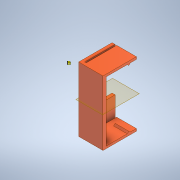
# Autodesk Inventor part: usbHubCaseTopChargingSide
Saved by Autodesk Inventor 2021.2 (Build 252289000, 289)
## iProperties
Created: 2021-02-17
Part Number: usbHubCaseTopChargingSide
Material: PC/ABS Plastic
Document SubType Name: Modeling
Designer: robst
Density: 0.357273 g/cm^3
Appearance: Smooth - Light Orange
Author: robst
Autodesk Inventor part; units mm, degrees
ref_plane "YZ Plane" through (0, 0, 0) normal (1, 0, 0) x (0, 1, 0)
ref_plane "XY Plane" through (0, 0, 0) normal (0, 0, 1) x (1, 0, 0)
sketch "Sketch1" plane through (0, 0, 0) normal (0, 0, 1) x (1, 0, 0)
  line L0 (-10.16, -26.9875) -> (10.16, -26.9875)
  line L1 (10.16, -26.9875) -> (10.16, 26.9875)
  line L2 (10.16, 26.9875) -> (-10.16, 26.9875)
  line L3 (-10.16, 26.9875) -> (-10.16, -26.9875)
  line L4 (-10.16, -26.9875) -> (10.16, 26.9875) construction
  line L5 (10.16, -26.9875) -> (-10.16, 26.9875) construction
  point P0 (0, 0)
  dimension "d0" = 53.975
  dimension "d1" = 20.32
  constraints: 12 end point, 2 midpoint, 2 parallel, 1 horizontal, 1 perpendicular
  measures "d0" distance of L2.end L0.start
  measures "d1" distance of L1.end L2.end
extrude "Extrusion1" add sketch "Sketch1" against normal blind 2.54
sketch "Sketch8" plane through (0, 0, -2.54) normal (0, 0, -1) x (-1, 0, 0)
  line L0 (-10.16, 26.9875) -> (-10.16, -26.9875) projected
  line L1 (10.16, -26.9875) -> (10.16, 26.9875) projected
  line L2 (-10.16, 26.9875) -> (10.16, 26.9875)
  line L3 (10.16, 26.9875) -> (10.16, 25.0825)
  line L4 (10.16, 25.0825) -> (-10.16, 25.0825)
  line L5 (-10.16, 25.0825) -> (-10.16, 26.9875)
  line L6 (-10.16, -26.9875) -> (10.16, -26.9875)
  line L7 (10.16, -26.9875) -> (10.16, -25.0825)
  line L8 (10.16, -25.0825) -> (-10.16, -25.0825)
  line L9 (-10.16, -25.0825) -> (-10.16, -26.9875)
  line L10 (10.16, 25.0825) -> (7.62, 25.0825)
  line L11 (7.62, 25.0825) -> (7.62, 9.525)
  line L12 (7.62, 9.525) -> (10.16, 9.525)
  line L13 (10.16, 9.525) -> (10.16, 25.0825)
  line L14 (10.16, -25.0825) -> (7.62, -25.0825)
  line L15 (7.62, -25.0825) -> (7.62, -9.525)
  line L16 (7.62, -9.525) -> (10.16, -9.525)
  line L17 (10.16, -9.525) -> (10.16, -25.0825)
  point P0 (0, 0)
  point P1 (10.16, -9.525)
  point P2 (10.16, 9.525)
  dimension "d32" = 1.905
  dimension "d33" = 1.905
  dimension "d34" = 2.54
  dimension "d35" = 15.5575
  dimension "d36" = 15.5575
  dimension "d37" = 2.54
  dimension "d54" = 19.05
  constraints: 32 end point, 8 parallel, 4 horizontal, 4 perpendicular, 2 point on line
  measures "d32" distance between parallel lines of L4 L2
  measures "d33" distance between parallel lines of L8 L6
  measures "d34" distance between parallel lines of L11 L1
  measures "d35" distance between parallel lines of L12 L4
  measures "d36" distance between parallel lines of L16 L8
  measures "d37" distance between parallel lines of L1 L15
  measures "d54" distance between parallel lines of L16 L12
extrude "Extrusion7" add sketch "Sketch8" along normal blind 25.4 contours L2 L1 L4 L0 | L8 L1 L6 L0 | L4 L1 L12 L11 | L15 L16 L1 L8
sketch "Sketch10" plane through (0, 0, -2.54) normal (0, 0, -1) x (-1, 0, 0)
  line L0 (7.62, 25.0825) -> (7.62, 9.525) projected
  line L1 (7.62, 9.525) -> (10.16, 9.525)
  line L2 (10.16, 9.525) -> (10.16, -9.525)
  line L3 (10.16, -9.525) -> (7.62, -9.525)
  line L4 (7.62, -9.525) -> (7.62, 9.525)
  point P0 (0, 0)
  constraints: 8 end point, 2 parallel, 1 horizontal, 1 perpendicular
extrude "Extrusion8" add sketch "Sketch10" along normal blind 6.096
sketch "Sketch11" plane through (10.16, -26.9875, 0) normal (1, 0, 0) x (0, 0, -1)
  line L0 (2.54, 1.905) -> (27.94, 1.905) projected
  line L1 (2.54, 52.07) -> (27.94, 52.07) projected
  line L2 (20.32, 1.905) -> (21.59, 3.175)
  line L3 (21.59, 3.175) -> (22.86, 1.905)
  line L4 (2.54, 1.905) -> (27.94, 1.905) projected
  line L5 (27.94, 17.4625) -> (27.94, 1.905) projected
  line L6 (20.32, 1.905) -> (22.86, 1.905)
  line L7 (0, 26.9875) -> (27.94, 26.9875) construction
  line L8 (2.54, 52.07) -> (27.94, 52.07)
  line L9 (20.32, 52.07) -> (21.59, 50.8)
  line L10 (21.59, 50.8) -> (22.86, 52.07)
  point P0 (22.86, 52.07)
  point P1 (20.32, 52.07)
  dimension "d42" = 90
  dimension "d43" = 135
  dimension "d44" = 1.27
  dimension "d45" = 6.35
  constraints: 14 end point, 3 point on line, 3 symmetric about line, 1 collinear, 1 horizontal
  measures "d42" angle of L3 L2
  measures "d43" angle of L3 L0
  measures "d44" distance from line of L2.end L0
  measures "d45" distance from line of L2.end L5
extrude "Extrusion9" add sketch "Sketch11" against normal up to surface (17.78 mm away)
sketch "Sketch12" plane through (-10.16, 26.9875, 0) normal (0, 1, 0) x (1, 0, 0)
  line L0 (2.54, 2.54) -> (2.54, 20.32) projected
  line L1 (2.54, 22.86) -> (2.54, 27.94) projected
  line L2 (2.54, 2.54) -> (20.32, 2.54) projected
  line L3 (2.54, 2.54) -> (3.81, 2.54)
  line L4 (3.81, 2.54) -> (3.81, 27.94)
  line L5 (3.81, 27.94) -> (2.54, 27.94)
  line L6 (2.54, 27.94) -> (2.54, 2.54)
  point P0 (10.16, 0)
  point P1 (2.54, 22.86)
  point P2 (2.54, 20.32)
  point P3 (3.81, 2.54)
  dimension "d48" = 1.27
  constraints: 8 end point, 2 parallel, 1 horizontal, 1 perpendicular
  measures "d48" distance between parallel lines of L1 L4
extrude "Extrusion10" cut sketch "Sketch12" against normal through all
sketch "Sketch16" plane through (0, 0, -2.54) normal (0, 0, -1) x (-1, 0, 0)
  line L0 (7.62, -9.525) -> (7.62, -26.9875) projected
  line L1 (-10.16, 25.0825) -> (-10.16, -25.0825) projected
  line L2 (-10.16, -26.9875) -> (6.35, -26.9875) projected
  line L3 (6.35, 26.9875) -> (-10.16, 26.9875) projected
  line L4 (-10.16, 26.9875) -> (10.16, 26.9875) construction
  line L5 (-0.762, 26.9875) -> (-0.762, -26.9875) construction
  line L6 (10.16, -26.9875) -> (-10.16, -26.9875) construction
  spline S0 degree 2 poles (-4.6934, -4.0246) (-4.4464, -4.0246) (-4.0018, -4.2006) (-3.8475, -4.358) knots 0 0 0 1 2 2 2
  spline S1 degree 2 poles (-3.8475, -4.358) (-3.6529, -4.5556) (-3.4523, -5.0898) (-3.4523, -5.4973) knots 0 0 0 1 2 2 2
  line L7 (-3.4523, -5.4973) -> (-3.4523, -5.9265)
  line L8 (-3.4523, -5.9265) -> (-2.032, -5.9265)
  line L9 (-2.032, -5.9265) -> (-2.032, -6.4328)
  line L10 (-2.032, -6.4328) -> (-5.842, -6.4328)
  line L11 (-5.842, -6.4328) -> (-5.842, -5.4757)
  spline S2 degree 2 poles (-5.842, -5.4757) (-5.842, -5.1361) (-5.7308, -4.6606) (-5.6043, -4.4784) knots 0 0 0 1 2 2 2
  spline S3 degree 2 poles (-5.6043, -4.4784) (-5.4591, -4.2654) (-5.0115, -4.0246) (-4.6934, -4.0246) knots 0 0 0 1 2 2 2
  spline S4 degree 2 poles (-4.678, -4.5525) (-4.8756, -4.5525) (-5.1658, -4.6884) (-5.2585, -4.8273) knots 0 0 0 1 2 2 2
  spline S5 degree 2 poles (-5.2585, -4.8273) (-5.3387, -4.9478) (-5.4036, -5.2689) (-5.4036, -5.5066) knots 0 0 0 1 2 2 2
  line L12 (-5.4036, -5.5066) -> (-5.4036, -5.9265)
  line L13 (-5.4036, -5.9265) -> (-3.8845, -5.9265)
  line L14 (-3.8845, -5.9265) -> (-3.8845, -5.5807)
  spline S6 degree 2 poles (-3.8845, -5.5807) (-3.8845, -5.2719) (-3.9833, -4.8922) (-4.113, -4.7687) knots 0 0 0 1 2 2 2
  spline S7 degree 2 poles (-4.113, -4.7687) (-4.2272, -4.6544) (-4.4958, -4.5525) (-4.678, -4.5525) knots 0 0 0 1 2 2 2
  line L15 (-5.842, -0.7796) -> (-2.032, -2.0918)
  line L16 (-2.032, -2.0918) -> (-2.032, -2.6383)
  line L17 (-2.032, -2.6383) -> (-5.842, -3.9505)
  line L18 (-5.842, -3.9505) -> (-5.842, -3.4071)
  line L19 (-5.842, -3.4071) -> (-2.6773, -2.3511)
  line L20 (-2.6773, -2.3511) -> (-5.842, -1.2952)
  line L21 (-5.842, -1.2952) -> (-5.842, -0.7796)
  line L22 (-3.4677, 0.9154) -> (-3.4677, -0.5264)
  line L23 (-3.4677, -0.5264) -> (-3.9308, -0.5264)
  line L24 (-3.9308, -0.5264) -> (-3.9308, 0.9154)
  line L25 (-3.9308, 0.9154) -> (-3.4677, 0.9154)
  spline S8 degree 2 poles (-3.937, 3.793) (-2.9119, 3.793) (-1.9517, 3.1971) (-1.9517, 2.5765) knots 0 0 0 1 2 2 2
  spline S9 degree 2 poles (-1.9517, 2.5765) (-1.9517, 1.9467) (-2.9305, 1.357) (-3.9339, 1.357) knots 0 0 0 1 2 2 2
  spline S10 degree 2 poles (-3.9339, 1.357) (-4.9651, 1.357) (-5.9192, 1.9529) (-5.9192, 2.5765) knots 0 0 0 1 2 2 2
  spline S11 degree 2 poles (-5.9192, 2.5765) (-5.9192, 3.2033) (-4.9312, 3.793) (-3.937, 3.793) knots 0 0 0 1 2 2 2
  spline S12 degree 2 poles (-2.7761, 3.1385) (-2.9644, 3.2126) (-3.5449, 3.2743) (-3.937, 3.2743) knots 0 0 0 1 2 2 2
  spline S13 degree 2 poles (-3.937, 3.2743) (-4.3291, 3.2743) (-4.9065, 3.2126) (-5.101, 3.1354) knots 0 0 0 1 2 2 2
  spline S14 degree 2 poles (-5.101, 3.1354) (-5.2955, 3.0582) (-5.4962, 2.7896) (-5.4962, 2.5765) knots 0 0 0 1 2 2 2
  spline S15 degree 2 poles (-5.4962, 2.5765) (-5.4962, 2.3635) (-5.2955, 2.0887) (-5.0948, 2.0084) knots 0 0 0 1 2 2 2
  spline S16 degree 2 poles (-5.0948, 2.0084) (-4.9003, 1.9312) (-4.3075, 1.8757) (-3.9339, 1.8757) knots 0 0 0 1 2 2 2
  spline S17 degree 2 poles (-3.9339, 1.8757) (-3.5325, 1.8757) (-2.9953, 1.9251) (-2.7854, 2.0053) knots 0 0 0 1 2 2 2
  spline S18 degree 2 poles (-2.7854, 2.0053) (-2.5878, 2.0794) (-2.3747, 2.3542) (-2.3747, 2.5765) knots 0 0 0 1 2 2 2
  spline S19 degree 2 poles (-2.3747, 2.5765) (-2.3747, 2.7865) (-2.5754, 3.0613) (-2.7761, 3.1385) knots 0 0 0 1 2 2 2
  line L26 (-3.3411, 6.7323) -> (-3.3411, 6.2785)
  line L27 (-3.3411, 6.2785) -> (-2.032, 6.2785)
  line L28 (-2.032, 6.2785) -> (-2.032, 5.7876)
  line L29 (-2.032, 5.7876) -> (-3.3411, 5.7876)
  line L30 (-3.3411, 5.7876) -> (-3.3411, 4.1049)
  line L31 (-3.3411, 4.1049) -> (-3.8783, 4.1049)
  line L32 (-3.8783, 4.1049) -> (-5.842, 5.8092)
  line L33 (-5.842, 5.8092) -> (-5.842, 6.2785)
  line L34 (-5.842, 6.2785) -> (-3.7517, 6.2785)
  line L35 (-3.7517, 6.2785) -> (-3.7517, 6.7323)
  line L36 (-3.7517, 6.7323) -> (-3.3411, 6.7323)
  line L37 (-3.7517, 5.7876) -> (-5.2399, 5.7876)
  line L38 (-5.2399, 5.7876) -> (-3.7517, 4.5062)
  line L39 (-3.7517, 4.5062) -> (-3.7517, 5.7876)
  spline S20 degree 2 poles (4.4171, -14.1378) (4.4171, -14.5083) (4.1671, -15.135) (3.917, -15.3635) knots 0 0 0 1 2 2 2
  spline S21 degree 2 poles (3.917, -15.3635) (3.67, -15.592) (2.929, -15.8421) (2.4473, -15.8421) knots 0 0 0 1 2 2 2
  spline S22 degree 2 poles (2.4473, -15.8421) (1.9687, -15.8421) (1.2586, -15.5982) (0.9962, -15.3666) knots 0 0 0 1 2 2 2
  spline S23 degree 2 poles (0.9962, -15.3666) (0.7399, -15.1381) (0.4713, -14.5144) (0.4713, -14.1285) knots 0 0 0 1 2 2 2
  spline S24 degree 2 poles (0.4713, -14.1285) (0.4713, -13.9371) (0.5269, -13.6005) (0.5701, -13.4585) knots 0 0 0 1 2 2 2
  spline S25 degree 2 poles (0.5701, -13.4585) (0.6102, -13.335) (0.7245, -13.0787) (0.7924, -12.9521) knots 0 0 0 1 2 2 2
  line L40 (0.7924, -12.9521) -> (1.4037, -12.9521)
  line L41 (1.4037, -12.9521) -> (1.4037, -12.9923)
  spline S26 degree 2 poles (1.4037, -12.9923) (1.342, -13.0602) (1.1691, -13.2702) (1.0857, -13.4215) knots 0 0 0 1 2 2 2
  spline S27 degree 2 poles (1.0857, -13.4215) (1.0054, -13.5666) (0.9035, -13.9093) (0.9035, -14.1316) knots 0 0 0 1 2 2 2
  spline S28 degree 2 poles (0.9035, -14.1316) (0.9035, -14.3755) (1.1042, -14.8108) (1.2957, -14.9745) knots 0 0 0 1 2 2 2
  spline S29 degree 2 poles (1.2957, -14.9745) (1.4902, -15.135) (2.0799, -15.3141) (2.4473, -15.3141) knots 0 0 0 1 2 2 2
  spline S30 degree 2 poles (2.4473, -15.3141) (2.8394, -15.3141) (3.4044, -15.1258) (3.5989, -14.9621) knots 0 0 0 1 2 2 2
  spline S31 degree 2 poles (3.5989, -14.9621) (3.7873, -14.8016) (3.9787, -14.3724) (3.9787, -14.1316) knots 0 0 0 1 2 2 2
  spline S32 degree 2 poles (3.9787, -14.1316) (3.9787, -13.9124) (3.8707, -13.5388) (3.7904, -13.3937) knots 0 0 0 1 2 2 2
  spline S33 degree 2 poles (3.7904, -13.3937) (3.7101, -13.2547) (3.5434, -13.0479) (3.4847, -12.9892) knots 0 0 0 1 2 2 2
  line L42 (3.4847, -12.9892) -> (3.4847, -12.9521)
  line L43 (3.4847, -12.9521) -> (4.0899, -12.9521)
  spline S34 degree 2 poles (4.0899, -12.9521) (4.1485, -13.0787) (4.2566, -13.301) (4.306, -13.4585) knots 0 0 0 1 2 2 2
  spline S35 degree 2 poles (4.306, -13.4585) (4.3616, -13.6252) (4.4171, -13.9093) (4.4171, -14.1378) knots 0 0 0 1 2 2 2
  line L44 (4.3492, -10.2722) -> (4.3492, -10.7538)
  line L45 (4.3492, -10.7538) -> (2.719, -10.7538)
  spline S36 degree 2 poles (2.719, -10.7538) (2.5214, -10.7538) (2.1818, -10.7909) (2.0799, -10.8465) knots 0 0 0 1 2 2 2
  spline S37 degree 2 poles (2.0799, -10.8465) (1.9718, -10.9051) (1.8669, -11.1151) (1.8669, -11.2941) knots 0 0 0 1 2 2 2
  spline S38 degree 2 poles (1.8669, -11.2941) (1.8669, -11.4732) (2.0583, -11.853) (2.2127, -12.0352) knots 0 0 0 1 2 2 2
  line L46 (2.2127, -12.0352) -> (4.3492, -12.0352)
  line L47 (4.3492, -12.0352) -> (4.3492, -12.5168)
  line L48 (4.3492, -12.5168) -> (0.3694, -12.5168)
  line L49 (0.3694, -12.5168) -> (0.3694, -12.0352)
  line L50 (0.3694, -12.0352) -> (1.8082, -12.0352)
  spline S39 degree 2 poles (1.8082, -12.0352) (1.6137, -11.819) (1.4099, -11.4022) (1.4099, -11.1676) knots 0 0 0 1 2 2 2
  spline S40 degree 2 poles (1.4099, -11.1676) (1.4099, -10.7477) (1.9657, -10.2722) (2.4936, -10.2722) knots 0 0 0 1 2 2 2
  line L51 (2.4936, -10.2722) -> (4.3492, -10.2722)
  spline S41 degree 2 poles (4.0466, -8.0029) (4.0899, -8.0615) (4.2442, -8.2591) (4.2906, -8.3517) knots 0 0 0 1 2 2 2
  spline S42 degree 2 poles (4.2906, -8.3517) (4.3585, -8.4783) (4.4295, -8.7161) (4.4295, -8.9322) knots 0 0 0 1 2 2 2
  spline S43 degree 2 poles (4.4295, -8.9322) (4.4295, -9.1082) (4.2967, -9.4262) (4.1763, -9.5466) knots 0 0 0 1 2 2 2
  spline S44 degree 2 poles (4.1763, -9.5466) (4.059, -9.6609) (3.7132, -9.7998) (3.5218, -9.7998) knots 0 0 0 1 2 2 2
  spline S45 degree 2 poles (3.5218, -9.7998) (3.2254, -9.7998) (2.8055, -9.5497) (2.685, -9.278) knots 0 0 0 1 2 2 2
  spline S46 degree 2 poles (2.685, -9.278) (2.5739, -9.0372) (2.4905, -8.3826) (2.4689, -8.0029) knots 0 0 0 1 2 2 2
  line L52 (2.4689, -8.0029) -> (2.3763, -8.0029)
  spline S47 degree 2 poles (2.3763, -8.0029) (2.2096, -8.0029) (2.0027, -8.1047) (1.944, -8.1974) knots 0 0 0 1 2 2 2
  spline S48 degree 2 poles (1.944, -8.1974) (1.8854, -8.29) (1.8483, -8.5555) (1.8483, -8.6975) knots 0 0 0 1 2 2 2
  spline S49 degree 2 poles (1.8483, -8.6975) (1.8483, -8.8643) (1.9471, -9.315) (2.0428, -9.5404) knots 0 0 0 1 2 2 2
  line L53 (2.0428, -9.5404) -> (2.0428, -9.5682)
  line L54 (2.0428, -9.5682) -> (1.5519, -9.5682)
  spline S50 degree 2 poles (1.5519, -9.5682) (1.5149, -9.4355) (1.4222, -8.9384) (1.4222, -8.6945) knots 0 0 0 1 2 2 2
  spline S51 degree 2 poles (1.4222, -8.6945) (1.4222, -8.3981) (1.5149, -7.9936) (1.6353, -7.833) knots 0 0 0 1 2 2 2
  spline S52 degree 2 poles (1.6353, -7.833) (1.7526, -7.6756) (2.1262, -7.5212) (2.3948, -7.5212) knots 0 0 0 1 2 2 2
  line L55 (2.3948, -7.5212) -> (4.3492, -7.5212)
  line L56 (4.3492, -7.5212) -> (4.3492, -8.0029)
  line L57 (4.3492, -8.0029) -> (4.0466, -8.0029)
  line L58 (3.6453, -8.0029) -> (2.8518, -8.0029)
  spline S53 degree 2 poles (2.8518, -8.0029) (2.8672, -8.1758) (2.9197, -8.6975) (2.9691, -8.8612) knots 0 0 0 1 2 2 2
  spline S54 degree 2 poles (2.9691, -8.8612) (3.0278, -9.0526) (3.2717, -9.3027) (3.4878, -9.3027) knots 0 0 0 1 2 2 2
  spline S55 degree 2 poles (3.4878, -9.3027) (3.7348, -9.3027) (3.9849, -9.0248) (3.9849, -8.7593) knots 0 0 0 1 2 2 2
  spline S56 degree 2 poles (3.9849, -8.7593) (3.9849, -8.5339) (3.7904, -8.1634) (3.6453, -8.0029) knots 0 0 0 1 2 2 2
  line L59 (2.0058, -5.3291) -> (2.0058, -5.3538)
  spline S57 degree 2 poles (2.0058, -5.3538) (1.9904, -5.4093) (1.9842, -5.5297) (1.9842, -5.6131) knots 0 0 0 1 2 2 2
  spline S58 degree 2 poles (1.9842, -5.6131) (1.9842, -5.8076) (2.154, -6.1905) (2.3207, -6.3634) knots 0 0 0 1 2 2 2
  line L60 (2.3207, -6.3634) -> (4.3492, -6.3634)
  line L61 (4.3492, -6.3634) -> (4.3492, -6.845)
  line L62 (4.3492, -6.845) -> (1.4902, -6.845)
  line L63 (1.4902, -6.845) -> (1.4902, -6.3634)
  line L64 (1.4902, -6.3634) -> (1.9163, -6.3634)
  spline S59 degree 2 poles (1.9163, -6.3634) (1.6816, -6.1009) (1.4902, -5.7088) (1.4902, -5.5236) knots 0 0 0 1 2 2 2
  spline S60 degree 2 poles (1.4902, -5.5236) (1.4902, -5.4495) (1.4963, -5.3754) (1.5056, -5.3291) knots 0 0 0 1 2 2 2
  line L65 (1.5056, -5.3291) -> (2.0058, -5.3291)
  spline S61 degree 2 poles (4.8062, -4.8536) (4.8278, -4.8042) (4.8957, -4.6158) (4.9235, -4.4954) knots 0 0 0 1 2 2 2
  spline S62 degree 2 poles (4.9235, -4.4954) (4.9575, -4.3627) (4.9976, -4.1373) (4.9976, -4.0045) knots 0 0 0 1 2 2 2
  spline S63 degree 2 poles (4.9976, -4.0045) (4.9976, -3.7822) (4.8803, -3.4735) (4.7753, -3.387) knots 0 0 0 1 2 2 2
  spline S64 degree 2 poles (4.7753, -3.387) (4.6703, -3.3036) (4.3955, -3.2388) (4.2195, -3.2388) knots 0 0 0 1 2 2 2
  line L66 (4.2195, -3.2388) -> (3.9695, -3.2388)
  spline S65 degree 2 poles (3.9695, -3.2388) (4.1393, -3.4333) (4.2998, -3.8069) (4.2998, -4.0879) knots 0 0 0 1 2 2 2
  spline S66 degree 2 poles (4.2998, -4.0879) (4.2998, -4.5757) (3.5742, -5.1531) (2.8919, -5.1531) knots 0 0 0 1 2 2 2
  spline S67 degree 2 poles (2.8919, -5.1531) (2.5368, -5.1531) (1.9873, -4.9524) (1.7928, -4.7857) knots 0 0 0 1 2 2 2
  spline S68 degree 2 poles (1.7928, -4.7857) (1.6106, -4.6251) (1.4099, -4.1836) (1.4099, -3.9489) knots 0 0 0 1 2 2 2
  spline S69 degree 2 poles (1.4099, -3.9489) (1.4099, -3.7266) (1.5149, -3.4024) (1.6106, -3.2388) knots 0 0 0 1 2 2 2
  line L67 (1.6106, -3.2388) -> (1.4902, -3.211)
  line L68 (1.4902, -3.211) -> (1.4902, -2.7572)
  line L69 (1.4902, -2.7572) -> (4.0219, -2.7572)
  spline S70 degree 2 poles (4.0219, -2.7572) (4.7506, -2.7572) (5.4298, -3.3901) (5.4298, -4.0416) knots 0 0 0 1 2 2 2
  spline S71 degree 2 poles (5.4298, -4.0416) (5.4298, -4.2515) (5.3619, -4.6899) (5.3063, -4.8783) knots 0 0 0 1 2 2 2
  line L70 (5.3063, -4.8783) -> (4.8062, -4.8783)
  line L71 (4.8062, -4.8783) -> (4.8062, -4.8536)
  line L72 (3.5742, -3.2388) -> (2.0027, -3.2388)
  spline S72 degree 2 poles (2.0027, -3.2388) (1.9163, -3.4179) (1.8422, -3.7205) (1.8422, -3.8718) knots 0 0 0 1 2 2 2
  spline S73 degree 2 poles (1.8422, -3.8718) (1.8422, -4.2361) (2.3794, -4.656) (2.8826, -4.656) knots 0 0 0 1 2 2 2
  spline S74 degree 2 poles (2.8826, -4.656) (3.3581, -4.656) (3.8552, -4.338) (3.8552, -3.9798) knots 0 0 0 1 2 2 2
  spline S75 degree 2 poles (3.8552, -3.9798) (3.8552, -3.7915) (3.707, -3.3963) (3.5742, -3.2388) knots 0 0 0 1 2 2 2
  line L73 (4.3492, -1.5685) -> (4.3492, -2.0501)
  line L74 (4.3492, -2.0501) -> (1.4902, -2.0501)
  line L75 (1.4902, -2.0501) -> (1.4902, -1.5685)
  line L76 (1.4902, -1.5685) -> (4.3492, -1.5685)
  line L77 (1.0147, -1.5345) -> (1.0147, -2.081)
  line L78 (1.0147, -2.081) -> (0.5145, -2.081)
  line L79 (0.5145, -2.081) -> (0.5145, -1.5345)
  line L80 (0.5145, -1.5345) -> (1.0147, -1.5345)
  line L81 (4.3492, 1.3832) -> (4.3492, 0.9016)
  line L82 (4.3492, 0.9016) -> (2.719, 0.9016)
  spline S76 degree 2 poles (2.719, 0.9016) (2.5214, 0.9016) (2.1818, 0.8645) (2.0799, 0.8089) knots 0 0 0 1 2 2 2
  spline S77 degree 2 poles (2.0799, 0.8089) (1.9718, 0.7503) (1.8669, 0.5403) (1.8669, 0.3612) knots 0 0 0 1 2 2 2
  spline S78 degree 2 poles (1.8669, 0.3612) (1.8669, 0.1822) (2.0583, -0.1976) (2.2127, -0.3798) knots 0 0 0 1 2 2 2
  line L83 (2.2127, -0.3798) -> (4.3492, -0.3798)
  line L84 (4.3492, -0.3798) -> (4.3492, -0.8614)
  line L85 (4.3492, -0.8614) -> (1.4902, -0.8614)
  line L86 (1.4902, -0.8614) -> (1.4902, -0.3798)
  line L87 (1.4902, -0.3798) -> (1.8082, -0.3798)
  spline S79 degree 2 poles (1.8082, -0.3798) (1.6137, -0.1636) (1.4099, 0.2532) (1.4099, 0.4878) knots 0 0 0 1 2 2 2
  spline S80 degree 2 poles (1.4099, 0.4878) (1.4099, 0.9077) (1.9657, 1.3832) (2.4936, 1.3832) knots 0 0 0 1 2 2 2
  line L88 (2.4936, 1.3832) -> (4.3492, 1.3832)
  spline S81 degree 2 poles (4.8062, 2.1613) (4.8278, 2.2107) (4.8957, 2.399) (4.9235, 2.5194) knots 0 0 0 1 2 2 2
  spline S82 degree 2 poles (4.9235, 2.5194) (4.9575, 2.6522) (4.9976, 2.8776) (4.9976, 3.0103) knots 0 0 0 1 2 2 2
  spline S83 degree 2 poles (4.9976, 3.0103) (4.9976, 3.2326) (4.8803, 3.5414) (4.7753, 3.6278) knots 0 0 0 1 2 2 2
  spline S84 degree 2 poles (4.7753, 3.6278) (4.6703, 3.7112) (4.3955, 3.776) (4.2195, 3.776) knots 0 0 0 1 2 2 2
  line L89 (4.2195, 3.776) -> (3.9695, 3.776)
  spline S85 degree 2 poles (3.9695, 3.776) (4.1393, 3.5815) (4.2998, 3.2079) (4.2998, 2.927) knots 0 0 0 1 2 2 2
  spline S86 degree 2 poles (4.2998, 2.927) (4.2998, 2.4391) (3.5742, 1.8618) (2.8919, 1.8618) knots 0 0 0 1 2 2 2
  spline S87 degree 2 poles (2.8919, 1.8618) (2.5368, 1.8618) (1.9873, 2.0625) (1.7928, 2.2292) knots 0 0 0 1 2 2 2
  spline S88 degree 2 poles (1.7928, 2.2292) (1.6106, 2.3897) (1.4099, 2.8313) (1.4099, 3.0659) knots 0 0 0 1 2 2 2
  spline S89 degree 2 poles (1.4099, 3.0659) (1.4099, 3.2882) (1.5149, 3.6124) (1.6106, 3.776) knots 0 0 0 1 2 2 2
  line L90 (1.6106, 3.776) -> (1.4902, 3.8038)
  line L91 (1.4902, 3.8038) -> (1.4902, 4.2577)
  line L92 (1.4902, 4.2577) -> (4.0219, 4.2577)
  spline S90 degree 2 poles (4.0219, 4.2577) (4.7506, 4.2577) (5.4298, 3.6247) (5.4298, 2.9733) knots 0 0 0 1 2 2 2
  spline S91 degree 2 poles (5.4298, 2.9733) (5.4298, 2.7633) (5.3619, 2.3249) (5.3063, 2.1366) knots 0 0 0 1 2 2 2
  line L93 (5.3063, 2.1366) -> (4.8062, 2.1366)
  line L94 (4.8062, 2.1366) -> (4.8062, 2.1613)
  line L95 (3.5742, 3.776) -> (2.0027, 3.776)
  spline S92 degree 2 poles (2.0027, 3.776) (1.9163, 3.597) (1.8422, 3.2944) (1.8422, 3.1431) knots 0 0 0 1 2 2 2
  spline S93 degree 2 poles (1.8422, 3.1431) (1.8422, 2.7788) (2.3794, 2.3589) (2.8826, 2.3589) knots 0 0 0 1 2 2 2
  spline S94 degree 2 poles (2.8826, 2.3589) (3.3581, 2.3589) (3.8552, 2.6769) (3.8552, 3.035) knots 0 0 0 1 2 2 2
  spline S95 degree 2 poles (3.8552, 3.035) (3.8552, 3.2234) (3.707, 3.6186) (3.5742, 3.776) knots 0 0 0 1 2 2 2
  spline S96 degree 2 poles (4.4171, 7.691) (4.4171, 7.2773) (4.2442, 6.6968) (4.1207, 6.4406) knots 0 0 0 1 2 2 2
  line L96 (4.1207, 6.4406) -> (3.4847, 6.4406)
  line L97 (3.4847, 6.4406) -> (3.4847, 6.4776)
  spline S97 degree 2 poles (3.4847, 6.4776) (3.7194, 6.7277) (3.9787, 7.3606) (3.9787, 7.654) knots 0 0 0 1 2 2 2
  spline S98 degree 2 poles (3.9787, 7.654) (3.9787, 8.0739) (3.6298, 8.503) (3.3427, 8.503) knots 0 0 0 1 2 2 2
  spline S99 degree 2 poles (3.3427, 8.503) (3.1142, 8.503) (2.8302, 8.2776) (2.7591, 8.0337) knots 0 0 0 1 2 2 2
  spline S100 degree 2 poles (2.7591, 8.0337) (2.7097, 7.8577) (2.6418, 7.5644) (2.5862, 7.3452) knots 0 0 0 1 2 2 2
  spline S101 degree 2 poles (2.5862, 7.3452) (2.5338, 7.1476) (2.3763, 6.8358) (2.2497, 6.7154) knots 0 0 0 1 2 2 2
  spline S102 degree 2 poles (2.2497, 6.7154) (2.1231, 6.598) (1.7835, 6.4684) (1.5612, 6.4684) knots 0 0 0 1 2 2 2
  spline S103 degree 2 poles (1.5612, 6.4684) (1.0981, 6.4684) (0.4713, 7.1908) (0.4713, 7.7497) knots 0 0 0 1 2 2 2
  spline S104 degree 2 poles (0.4713, 7.7497) (0.4713, 8.0708) (0.5979, 8.6389) (0.7183, 8.8828) knots 0 0 0 1 2 2 2
  line L98 (0.7183, 8.8828) -> (1.3234, 8.8828)
  line L99 (1.3234, 8.8828) -> (1.3234, 8.8457)
  spline S105 degree 2 poles (1.3234, 8.8457) (1.1567, 8.6636) (0.9097, 8.0955) (0.9097, 7.7836) knots 0 0 0 1 2 2 2
  spline S106 degree 2 poles (0.9097, 7.7836) (0.9097, 7.4317) (1.2401, 6.9963) (1.5087, 6.9963) knots 0 0 0 1 2 2 2
  spline S107 degree 2 poles (1.5087, 6.9963) (1.7495, 6.9963) (2.0367, 7.2526) (2.1015, 7.4934) knots 0 0 0 1 2 2 2
  spline S108 degree 2 poles (2.1015, 7.4934) (2.1447, 7.654) (2.2559, 8.1202) (2.3022, 8.2746) knots 0 0 0 1 2 2 2
  spline S109 degree 2 poles (2.3022, 8.2746) (2.4226, 8.6667) (2.9073, 9.031) (3.2624, 9.031) knots 0 0 0 1 2 2 2
  spline S110 degree 2 poles (3.2624, 9.031) (3.4878, 9.031) (3.9201, 8.8488) (4.0713, 8.6852) knots 0 0 0 1 2 2 2
  spline S111 degree 2 poles (4.0713, 8.6852) (4.2381, 8.503) (4.4171, 8.0399) (4.4171, 7.691) knots 0 0 0 1 2 2 2
  line L100 (4.3492, 10.0005) -> (4.3492, 9.5188)
  line L101 (4.3492, 9.5188) -> (1.4902, 9.5188)
  line L102 (1.4902, 9.5188) -> (1.4902, 10.0005)
  line L103 (1.4902, 10.0005) -> (4.3492, 10.0005)
  line L104 (1.0147, 10.0344) -> (1.0147, 9.4879)
  line L105 (1.0147, 9.4879) -> (0.5145, 9.4879)
  line L106 (0.5145, 9.4879) -> (0.5145, 10.0344)
  line L107 (0.5145, 10.0344) -> (1.0147, 10.0344)
  line L108 (4.3492, 12.9058) -> (4.3492, 12.4242)
  line L109 (4.3492, 12.4242) -> (4.059, 12.4242)
  spline S112 degree 2 poles (4.059, 12.4242) (4.1516, 12.313) (4.2751, 12.1494) (4.3276, 12.0382) knots 0 0 0 1 2 2 2
  spline S113 degree 2 poles (4.3276, 12.0382) (4.377, 11.9364) (4.4295, 11.7171) (4.4295, 11.572) knots 0 0 0 1 2 2 2
  spline S114 degree 2 poles (4.4295, 11.572) (4.4295, 11.3374) (4.235, 10.9422) (4.0466, 10.8032) knots 0 0 0 1 2 2 2
  spline S115 degree 2 poles (4.0466, 10.8032) (3.8583, 10.6643) (3.3025, 10.5099) (2.9413, 10.5099) knots 0 0 0 1 2 2 2
  spline S116 degree 2 poles (2.9413, 10.5099) (2.5646, 10.5099) (2.0151, 10.7044) (1.8082, 10.8742) knots 0 0 0 1 2 2 2
  spline S117 degree 2 poles (1.8082, 10.8742) (1.6229, 11.0317) (1.4099, 11.4732) (1.4099, 11.7171) knots 0 0 0 1 2 2 2
  spline S118 degree 2 poles (1.4099, 11.7171) (1.4099, 11.9302) (1.5056, 12.2482) (1.6044, 12.4242) knots 0 0 0 1 2 2 2
  line L110 (1.6044, 12.4242) -> (0.3694, 12.4242)
  line L111 (0.3694, 12.4242) -> (0.3694, 12.9058)
  line L112 (0.3694, 12.9058) -> (4.3492, 12.9058)
  line L113 (3.6545, 12.4242) -> (2.0027, 12.4242)
  spline S119 degree 2 poles (2.0027, 12.4242) (1.9163, 12.2451) (1.8514, 11.9611) (1.8514, 11.7974) knots 0 0 0 1 2 2 2
  spline S120 degree 2 poles (1.8514, 11.7974) (1.8514, 11.4269) (2.4072, 11.007) (2.932, 11.007) knots 0 0 0 1 2 2 2
  spline S121 degree 2 poles (2.932, 11.007) (3.4384, 11.007) (3.9725, 11.3281) (3.9725, 11.6832) knots 0 0 0 1 2 2 2
  spline S122 degree 2 poles (3.9725, 11.6832) (3.9725, 11.8715) (3.7996, 12.2544) (3.6545, 12.4242) knots 0 0 0 1 2 2 2
  spline S123 degree 2 poles (4.4141, 14.8448) (4.4141, 14.1594) (3.6453, 13.406) (2.9351, 13.406) knots 0 0 0 1 2 2 2
  spline S124 degree 2 poles (2.9351, 13.406) (2.2374, 13.406) (1.4099, 14.1378) (1.4099, 14.7275) knots 0 0 0 1 2 2 2
  spline S125 degree 2 poles (1.4099, 14.7275) (1.4099, 14.993) (1.5643, 15.4036) (1.7279, 15.5549) knots 0 0 0 1 2 2 2
  spline S126 degree 2 poles (1.7279, 15.5549) (1.8916, 15.7093) (2.3639, 15.8729) (2.7067, 15.8729) knots 0 0 0 1 2 2 2
  line L114 (2.7067, 15.8729) -> (2.9691, 15.8729)
  line L115 (2.9691, 15.8729) -> (2.9691, 13.8938)
  spline S127 degree 2 poles (2.9691, 13.8938) (3.4662, 13.8938) (3.9942, 14.394) (3.9942, 14.8386) knots 0 0 0 1 2 2 2
  spline S128 degree 2 poles (3.9942, 14.8386) (3.9942, 14.9961) (3.9231, 15.3018) (3.8676, 15.4253) knots 0 0 0 1 2 2 2
  spline S129 degree 2 poles (3.8676, 15.4253) (3.8058, 15.5549) (3.6978, 15.734) (3.6483, 15.7927) knots 0 0 0 1 2 2 2
  line L116 (3.6483, 15.7927) -> (3.6483, 15.8205)
  line L117 (3.6483, 15.8205) -> (4.1732, 15.8205)
  spline S130 degree 2 poles (4.1732, 15.8205) (4.2072, 15.7371) (4.306, 15.4839) (4.3338, 15.3851) knots 0 0 0 1 2 2 2
  spline S131 degree 2 poles (4.3338, 15.3851) (4.3739, 15.2462) (4.4141, 15.0177) (4.4141, 14.8448) knots 0 0 0 1 2 2 2
  spline S132 degree 2 poles (2.6017, 15.4036) (2.4072, 15.3975) (2.1231, 15.3172) (2.0274, 15.24) knots 0 0 0 1 2 2 2
  spline S133 degree 2 poles (2.0274, 15.24) (1.9193, 15.1566) (1.8051, 14.8942) (1.8051, 14.6997) knots 0 0 0 1 2 2 2
  spline S134 degree 2 poles (1.8051, 14.6997) (1.8051, 14.5083) (1.9193, 14.2396) (2.0305, 14.1285) knots 0 0 0 1 2 2 2
  spline S135 degree 2 poles (2.0305, 14.1285) (2.1447, 14.0204) (2.4195, 13.9093) (2.6017, 13.8938) knots 0 0 0 1 2 2 2
  line L118 (2.6017, 13.8938) -> (2.6017, 15.4036)
  point P0 (0, 0)
  dimension "d51" = 9.398
  constraints: 2 end point, 2 point on line, 1 perpendicular, 1 vertical
  measures "d51" distance between parallel lines of L5 L1
extrude "Extrusion11" cut sketch "Sketch16" against normal blind 1.27
sketch "Sketch17" plane through (10.16, 25.0825, -27.94) normal (0, -1, 0) x (1, 0, 0)
  line L0 (-17.78, 25.4) -> (-17.78, 0) projected
  line L1 (-17.78, 3.907) -> (-11.43, 3.907)
  line L2 (-11.43, 3.907) -> (-11.43, 9.1028)
  line L3 (-11.43, 9.1028) -> (-17.78, 9.1028)
  line L4 (-17.78, 9.1028) -> (-17.78, 3.907)
  point P0 (-10.16, 27.94)
  dimension "d55" = 6.35
  constraints: 8 end point, 2 parallel, 1 horizontal, 1 perpendicular, 1 point on line
  measures "d55" distance between parallel lines of L2 L0
extrude "Extrusion12" cut sketch "Sketch17" along normal blind 1.5875
mirror "Mirror1" about plane through (0, 0, 0) normal (0, 1, 0) of "Extrusion12"
equation "\"d2\" = usbHolderWallThickness"
equation "\"usbHolderWallThickness\" = 2.54"
equation "\"usbHubWidth\" = 44.45"
equation "\"usbHubDepth\" = 27.432"
equation "\"usbHubLength\" = 109.22"
equation "\"usbHolderWidth\" = 58.42"
equation "\"usbHolderLength\" = usbHubLength + 2 * usbHolderWallThickness"
equation "\"holePatternLength\" = 25.4"
equation "\"holePatternWidth\" = 50.8"
body "Solid1"
